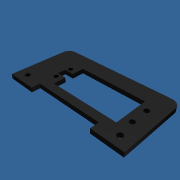
# Autodesk Inventor part: Acrylic_YawServoSupport_1
Saved by Autodesk Inventor 2012 (Build 160160000, 160)
## iProperties
Created: 2014-03-29
Part Number: Acrylic_YawServoSupport_1
Material: Default
Document SubType Name: Modeling
Designer: Admin
Density: 1 g/cm^3
Author: Admin
Autodesk Inventor part; units mm, degrees
ref_plane "YZ Plane" through (0, 0, 0) normal (1, 0, 0) x (0, 1, 0)
ref_plane "XZ Plane" through (0, 0, 0) normal (0, 1, 0) x (-1, 0, 0)
ref_plane "XY Plane" through (0, 0, 0) normal (0, 0, 1) x (1, 0, 0)
sketch "Sketch1" plane through (0, 0, 0) normal (0, 0, 1) x (1, 0, 0)
  line L0 (-53.9497, 0) -> (53.9497, 0) projected
  line L1 (0, -8.2071) -> (0, 49.2426) projected
  line L2 (-37.5, 0) -> (37.5, 0)
  line L3 (37.5, 0) -> (37.5, 35)
  line L4 (32.5, 40) -> (-32.5, 40)
  line L5 (-37.5, 35) -> (-37.5, 0)
  arc A0 (-32.5, 40) -> (-37.5, 35) centre (-32.5, 35) ccw
  arc A1 (37.5, 35) -> (32.5, 40) centre (32.5, 35) ccw
  point P0 (0, 0)
  point P1 (37.5, 40)
  point P2 (-37.5, 40)
  dimension "d0" = 75
  dimension "d1" = 40
  dimension "d2" = 37.5
  dimension "d5" = 5
  constraints: 8 end point, 5 point on line, 4 point on circle, 4 tangent, 2 centre point, 2 parallel, 1 equal radius, 1 horizontal, 1 perpendicular
  measures "d0" distance of point (-37.5, 40) point (37.5, 40)
  measures "d1" distance of point (37.5, 40) L2.end
  measures "d2" distance between parallel lines of L5 L1
  measures "d5" radius of A0
extrude "Extrusion1" add sketch "Sketch1" along normal blind 2.8
sketch "Sketch2" plane through (0, 0, 2.8) normal (0, 0, 1) x (1, 0, 0)
  line L0 (37.5, 0) -> (-37.5, 0) projected
  line L1 (37.5, 35) -> (37.5, 0) projected
  line L2 (-20, 0) -> (20, 0)
  line L3 (20, 0) -> (20, 5)
  line L4 (20, 5) -> (-20, 5)
  line L5 (-20, 5) -> (-20, 0)
  line L6 (-15.15, 22.4) -> (-15.15, 29.8)
  line L7 (-15.15, 29.8) -> (25.15, 29.8)
  line L8 (-21.15, 22.4) -> (-15.15, 22.4)
  line L9 (-21.15, 17.4) -> (-21.15, 22.4)
  line L10 (-15.15, 17.4) -> (-21.15, 17.4)
  line L11 (-15.15, 10) -> (-15.15, 17.4)
  line L12 (25.15, 10) -> (-15.15, 10)
  line L13 (25.15, 29.8) -> (25.15, 10)
  line L14 (-15.15, 29.8) -> (25.15, 29.8)
  point P0 (0, 0)
  dimension "d6" = 17.5
  dimension "d7" = 40
  constraints: 26 end point, 6 horizontal, 4 vertical, 2 parallel, 1 perpendicular, 1 point on line, 8 other
  measures "d6" distance between parallel lines of L1 L3
  measures "d7" distance of L3.end L4.end
extrude "Extrusion2" cut sketch "Sketch2" against normal blind 10
sketch "Sketch3" plane through (0, 0, 2.8) normal (0, 0, 1) x (1, 0, 0)
  circle A0 centre (-19.5, 24.9) radius 2.5
  circle A1 centre (-19.5, 14.9) radius 2.5
  circle A2 centre (29.5, 14.9) radius 2.5
  circle A3 centre (29.5, 24.9) radius 2.5
  circle A4 centre (29.5, 14.9) radius 1.5
  circle A5 centre (29.5, 24.9) radius 1.5
  circle A6 centre (-19.5, 14.9) radius 1.5
  circle A7 centre (-19.5, 24.9) radius 1.5
  line L0 (-15.15, 17.4) -> (-21.15, 17.4) projected
  line L1 (29.3, 5.4) -> (29.3, 7)
  line L2 (32.5, 7) -> (32.5, 3.8)
  line L3 (29.3, 3.8) -> (29.3, 5.4)
  arc A8 (29.3, 3.8) -> (32.5, 3.8) centre (30.9, 3.8) ccw
  arc A9 (32.5, 7) -> (29.3, 7) centre (30.9, 7) ccw
  line L4 (-15.15, 10) -> (-15.15, 17.4) projected
  line L5 (-32.5, 5.4) -> (-32.5, 7)
  line L6 (-29.3, 7) -> (-29.3, 3.8)
  line L7 (-32.5, 3.8) -> (-32.5, 5.4)
  arc A10 (-29.3, 7) -> (-32.5, 7) centre (-30.9, 7) ccw
  arc A11 (-32.5, 3.8) -> (-29.3, 3.8) centre (-30.9, 3.8) ccw
  point P0 (0, 0)
  dimension "d10" = 3
  dimension "d11" = 3
  dimension "d12" = 3
  dimension "d13" = 3
  constraints: 12 centre point, 12 end point, 8 point on circle, 4 coincident, 3 parallel, 2 collinear, 1 perpendicular, 8 other
  measures "d10" diameter of A4
  measures "d11" diameter of A5
  measures "d12" diameter of A6
  measures "d13" diameter of A7
extrude "Extrusion3" cut sketch "Sketch3" against normal through all contours A4 | A5 | A6 | A7 | L1 A9 L2 A8 L3 | L5 A10 L6 A11 L7
equation "\"d2\" = 0.5 * d0"
body "Solid1"
